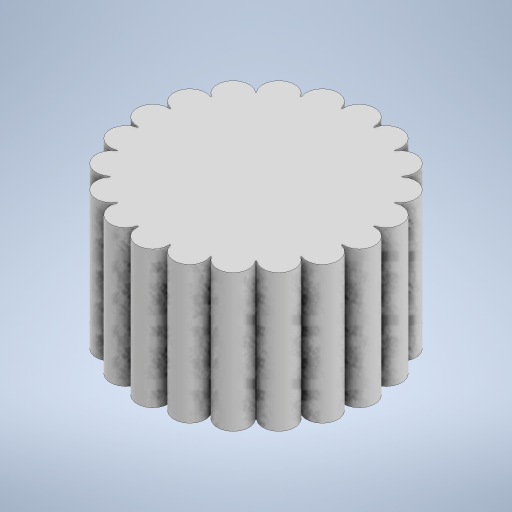
# Autodesk Inventor part: 책상 고정대 손잡이
Saved by Autodesk Inventor 2023 (Build 270158000, 158)
## iProperties
Created: 2022-11-11
Part Number: 책상 고정대 손잡이
Material: 일반
Document SubType Name: Modeling
Designer: hyunsu
Density: 1 g/cm^3
Appearance: 기본값
Author: hyunsu
Autodesk Inventor part; units mm, degrees
ref_plane "YZ Plane" through (0, 0, 0) normal (1, 0, 0) x (0, 1, 0)
ref_plane "XZ Plane" through (0, 0, 0) normal (0, 1, 0) x (-1, 0, 0)
ref_plane "XY Plane" through (0, 0, 0) normal (0, 0, 1) x (1, 0, 0)
sketch "스케치1" plane through (0, 0, 0) normal (0, 1, 0) x (-1, 0, 0)
  line L0 (4.5033, 0) -> (2.2517, -3.9)
  line L1 (2.2517, -3.9) -> (-2.2517, -3.9)
  line L2 (-2.2517, -3.9) -> (-4.5033, 0)
  line L3 (-4.5033, 0) -> (-2.2517, 3.9)
  line L4 (-2.2517, 3.9) -> (2.2517, 3.9)
  line L5 (2.2517, 3.9) -> (4.5033, 0)
  point P0 (0, 0)
  point P1 (0, 0)
  dimension "d0" = 7.8
  constraints: 12 end point, 1 coincident, 13 other
  measures "d0" distance between parallel lines of L1 L4
extrude "돌출1" add sketch "스케치1" against normal blind 5
sketch "스케치2" plane through (0, 0, 0) normal (0, 1, 0) x (1, 0, 0)
  circle A0 centre (0, 0) radius 8.25
  circle A1 centre (-9.75, 0) radius 1.5
  circle A2 centre (-9.2728, -3.0129) radius 1.5
  circle A3 centre (-7.8879, -5.7309) radius 1.5
  circle A4 centre (-5.7309, -7.8879) radius 1.5
  circle A5 centre (-3.0129, -9.2728) radius 1.5
  circle A6 centre (0, -9.75) radius 1.5
  circle A7 centre (3.0129, -9.2728) radius 1.5
  circle A8 centre (5.7309, -7.8879) radius 1.5
  circle A9 centre (7.8879, -5.7309) radius 1.5
  circle A10 centre (9.2728, -3.0129) radius 1.5
  circle A11 centre (9.75, 0) radius 1.5
  circle A12 centre (9.2728, 3.0129) radius 1.5
  circle A13 centre (7.8879, 5.7309) radius 1.5
  circle A14 centre (5.7309, 7.8879) radius 1.5
  circle A15 centre (3.0129, 9.2728) radius 1.5
  circle A16 centre (0, 9.75) radius 1.5
  circle A17 centre (-3.0129, 9.2728) radius 1.5
  circle A18 centre (-5.7309, 7.8879) radius 1.5
  circle A19 centre (-7.8879, 5.7309) radius 1.5
  circle A20 centre (-9.2728, 3.0129) radius 1.5
  circle A21 centre (0, 0) radius 9.75
  point P0 (9.6252, -1.5549)
  point P1 (9.6346, -1.4956)
  point P2 (9.6346, 1.4956)
  point P3 (9.6252, 1.5549)
  point P4 (8.7009, 4.3996)
  point P5 (8.6736, 4.4532)
  point P6 (6.9155, 6.873)
  point P7 (6.873, 6.9155)
  point P8 (4.4532, 8.6736)
  point P9 (4.3996, 8.7009)
  point P10 (1.5549, 9.6252)
  point P11 (1.4956, 9.6346)
  point P12 (-1.4956, 9.6346)
  point P13 (-1.5549, 9.6252)
  point P14 (-4.3996, 8.7009)
  point P15 (-4.4532, 8.6736)
  point P16 (-6.873, 6.9155)
  point P17 (-6.9155, 6.873)
  point P18 (-8.6736, 4.4532)
  point P19 (-8.7009, 4.3996)
  point P20 (-9.6252, 1.5549)
  point P21 (-9.6346, 1.4956)
  point P22 (-9.6346, -1.4956)
  point P23 (-9.6252, -1.5549)
  point P24 (-8.7009, -4.3996)
  point P25 (-8.6736, -4.4532)
  point P26 (-6.9155, -6.873)
  point P27 (-6.873, -6.9155)
  point P28 (-4.4532, -8.6736)
  point P29 (-4.3996, -8.7009)
  point P30 (-1.5549, -9.6252)
  point P31 (-1.4956, -9.6346)
  point P32 (1.4956, -9.6346)
  point P33 (1.5549, -9.6252)
  point P34 (4.3996, -8.7009)
  point P35 (4.4532, -8.6736)
  point P36 (6.873, -6.9155)
  point P37 (6.9155, -6.873)
  point P38 (8.6736, -4.4532)
  point P39 (8.7009, -4.3996)
  dimension "d3" = 16.5
  dimension "d4" = 3
  dimension "d7" = 360
  constraints: 21 centre point, 2 coincident, 1 horizontal alignment, 1 tangent, 44 other
  measures "d3" diameter of A0
  measures "d4" diameter of A1
extrude "돌출2" add sketch "스케치2" against normal blind 10 contours A11 A21 A10 A0 | A0 A12 A21 A11 | A11 A21 | A0 A13 A21 A12 | A12 A21 | A10 A21 A9 A0 | A10 A21 | A11 A21 | A0 A14 A21 A13 | A13 A21 | A12 A21 | A9 A21 A8 A0 | A9 A21 | A10 A21 | A0 A15 A21 A14 | A14 A21 | A13 A21 | A8 A21 A7 A0 | A8 A21 | A9 A21 | A0 A16 A21 A15 | A15 A21 | A14 A21 | A7 A21 A6 A0 | A7 A21 | A8 A21 | A0 A17 A21 A16 | A16 A21 | A15 A21 | A6 A21 A5 A0 | A6 A21 | A7 A21 | A0 A18 A21 A17 | A17 A21 | A16 A21 | A5 A21 A4 A0 | A5 A21 | A6 A21 | A0 A19 A21 A18 | A18 A21 | A17 A21 | A4 A21 A3 A0 | A4 A21 | A21 A5 | A0 A20 A21 A19 | A19 A21 | A18 A21 | A3 A21 A2 A0 | A3 A21 | A21 A4 | A0 A1 A21 A20 | A20 A21 | A19 A21 | A2 A21 A1 A0 | A2 A21 | A21 A3 | A1 A21 | A20 A21 | A21 A2 | A21 A1
sketch "스케치3" plane through (0, 0, 0) normal (0, 1, 0) x (1, 0, 0)
  arc A0 (9.6346, -1.4956) -> (9.6346, 1.4956) centre (9.75, 0) ccw projected
  arc A1 (9.6346, 1.4956) -> (9.6252, 1.5549) centre (0, 0) ccw projected
  arc A2 (9.6252, 1.5549) -> (8.7009, 4.3996) centre (9.2728, 3.0129) ccw projected
  arc A3 (8.7009, 4.3996) -> (8.6736, 4.4532) centre (0, 0) ccw projected
  arc A4 (8.6736, 4.4532) -> (6.9155, 6.873) centre (7.8879, 5.7309) ccw projected
  arc A5 (6.9155, 6.873) -> (6.873, 6.9155) centre (0, 0) ccw projected
  arc A6 (6.873, 6.9155) -> (4.4532, 8.6736) centre (5.7309, 7.8879) ccw projected
  arc A7 (4.4532, 8.6736) -> (4.3996, 8.7009) centre (0, 0) ccw projected
  arc A8 (4.3996, 8.7009) -> (1.5549, 9.6252) centre (3.0129, 9.2728) ccw projected
  arc A9 (1.5549, 9.6252) -> (1.4956, 9.6346) centre (0, 0) ccw projected
  arc A10 (1.4956, 9.6346) -> (-1.4956, 9.6346) centre (0, 9.75) ccw projected
  arc A11 (-1.4956, 9.6346) -> (-1.5549, 9.6252) centre (0, 0) ccw projected
  arc A12 (-1.5549, 9.6252) -> (-4.3996, 8.7009) centre (-3.0129, 9.2728) ccw projected
  arc A13 (-4.3996, 8.7009) -> (-4.4532, 8.6736) centre (0, 0) ccw projected
  arc A14 (-4.4532, 8.6736) -> (-6.873, 6.9155) centre (-5.7309, 7.8879) ccw projected
  arc A15 (-6.873, 6.9155) -> (-6.9155, 6.873) centre (0, 0) ccw projected
  arc A16 (-6.9155, 6.873) -> (-8.6736, 4.4532) centre (-7.8879, 5.7309) ccw projected
  arc A17 (-8.6736, 4.4532) -> (-8.7009, 4.3996) centre (0, 0) ccw projected
  arc A18 (-8.7009, 4.3996) -> (-9.6252, 1.5549) centre (-9.2728, 3.0129) ccw projected
  arc A19 (-9.6252, 1.5549) -> (-9.6346, 1.4956) centre (0, 0) ccw projected
  arc A20 (-9.6346, 1.4956) -> (-9.6346, -1.4956) centre (-9.75, 0) ccw projected
  arc A21 (-9.6346, -1.4956) -> (-9.6252, -1.5549) centre (0, 0) ccw projected
  arc A22 (-9.6252, -1.5549) -> (-8.7009, -4.3996) centre (-9.2728, -3.0129) ccw projected
  arc A23 (-8.7009, -4.3996) -> (-8.6736, -4.4532) centre (0, 0) ccw projected
  arc A24 (-8.6736, -4.4532) -> (-6.9155, -6.873) centre (-7.8879, -5.7309) ccw projected
  arc A25 (-6.9155, -6.873) -> (-6.873, -6.9155) centre (0, 0) ccw projected
  arc A26 (-6.873, -6.9155) -> (-4.4532, -8.6736) centre (-5.7309, -7.8879) ccw projected
  arc A27 (-4.4532, -8.6736) -> (-4.3996, -8.7009) centre (0, 0) ccw projected
  arc A28 (-4.3996, -8.7009) -> (-1.5549, -9.6252) centre (-3.0129, -9.2728) ccw projected
  arc A29 (-1.5549, -9.6252) -> (-1.4956, -9.6346) centre (0, 0) ccw projected
  arc A30 (-1.4956, -9.6346) -> (1.4956, -9.6346) centre (0, -9.75) ccw projected
  arc A31 (1.4956, -9.6346) -> (1.5549, -9.6252) centre (0, 0) ccw projected
  arc A32 (1.5549, -9.6252) -> (4.3996, -8.7009) centre (3.0129, -9.2728) ccw projected
  arc A33 (4.3996, -8.7009) -> (4.4532, -8.6736) centre (0, 0) ccw projected
  arc A34 (4.4532, -8.6736) -> (6.873, -6.9155) centre (5.7309, -7.8879) ccw projected
  arc A35 (6.873, -6.9155) -> (6.9155, -6.873) centre (0, 0) ccw projected
  arc A36 (6.9155, -6.873) -> (8.6736, -4.4532) centre (7.8879, -5.7309) ccw projected
  arc A37 (8.6736, -4.4532) -> (8.7009, -4.3996) centre (0, 0) ccw projected
  arc A38 (8.7009, -4.3996) -> (9.6252, -1.5549) centre (9.2728, -3.0129) ccw projected
  arc A39 (9.6252, -1.5549) -> (9.6346, -1.4956) centre (0, 0) ccw projected
  circle A40 centre (0, 0) radius 8.25 construction
extrude "돌출3" add sketch "스케치3" along normal blind 3
